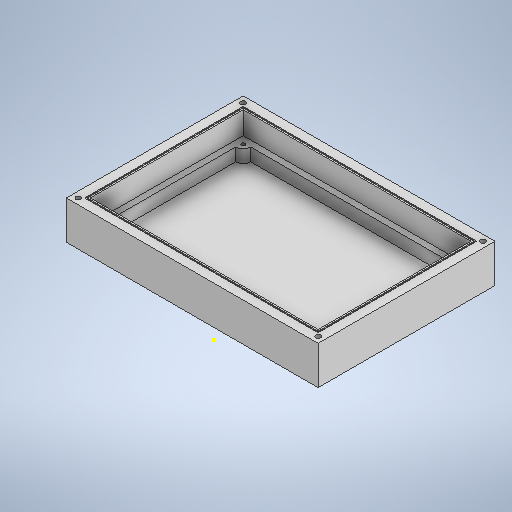
# Autodesk Inventor part: peça pi2
Saved by Autodesk Inventor 2025.1 (Build 291241000, 241)
## iProperties
Created: 2024-10-30
Part Number: peça pi2
Material: Genérico
Document SubType Name: Modeling
Designer: Willi
Density: 1 g/cm^3
Appearance: Padrão
Author: Willi
Autodesk Inventor part; units mm, degrees
ref_plane "YZ Plane" through (0, 0, 0) normal (1, 0, 0) x (0, 1, 0)
ref_plane "XZ Plane" through (0, 0, 0) normal (0, 1, 0) x (-1, 0, 0)
ref_plane "XY Plane" through (0, 0, 0) normal (0, 0, 1) x (1, 0, 0)
sketch "Esboço9" plane through (0, 0, 0) normal (0, 1, 0) x (-1, 0, 0)
  line L0 (123.7607, -142.906) -> (-28.2393, -142.906)
  line L1 (-28.2393, -142.906) -> (-28.2393, -40.906)
  line L2 (-28.2393, -40.906) -> (123.7607, -40.906)
  line L3 (123.7607, -40.906) -> (123.7607, -142.906)
  point P0 (0, 0)
  dimension "d42" = 152
  dimension "d43" = 102
  constraints: 8 end point, 2 parallel, 1 horizontal, 1 perpendicular
  measures "d42" distance of L1.end L2.end
  measures "d43" distance of L0.end L1.end
extrude "Extrusão7" add sketch "Esboço9" along normal blind 10.6
shell "Casca2" thickness 2 removed faces 1 at (-22.4273, 10.6, -74.906)
sketch "Esboço10" plane through (0, 10.6, 0) normal (0, 1, 0) x (1, 0, 0)
  line L0 (-123.7607, 142.906) -> (-123.7607, 40.906) projected
  line L1 (-123.7607, 40.906) -> (28.2393, 40.906) projected
  line L2 (28.2393, 142.906) -> (-123.7607, 142.906) projected
  line L3 (28.2393, 40.906) -> (28.2393, 142.906) projected
  line L4 (-123.7607, 40.906) -> (-131.7607, 40.906)
  line L5 (-131.7607, 40.906) -> (-131.7607, 142.906)
  line L6 (-131.7607, 142.906) -> (-123.7607, 142.906)
  line L7 (-123.7607, 142.906) -> (-123.7607, 40.906)
  line L8 (-131.7607, 142.906) -> (28.2393, 142.906)
  line L9 (28.2393, 142.906) -> (28.2393, 150.906)
  line L10 (28.2393, 150.906) -> (-131.7607, 150.906)
  line L11 (-131.7607, 150.906) -> (-131.7607, 142.906)
  line L12 (28.2393, 40.906) -> (36.2393, 40.906)
  line L13 (36.2393, 40.906) -> (36.2393, 150.906)
  line L14 (36.2393, 150.906) -> (28.2393, 150.906)
  line L15 (28.2393, 150.906) -> (28.2393, 40.906)
  line L16 (-131.7607, 40.906) -> (36.2393, 40.906)
  line L17 (36.2393, 40.906) -> (36.2393, 32.906)
  line L18 (36.2393, 32.906) -> (-131.7607, 32.906)
  line L19 (-131.7607, 32.906) -> (-131.7607, 40.906)
  point P0 (0, 0)
  dimension "d47" = 8
  dimension "d48" = 8
  dimension "d49" = 8
  dimension "d50" = 8
  constraints: 32 end point, 8 parallel, 4 horizontal, 4 perpendicular, 2 point on line
  measures "d47" distance of L5.end L6.end
  measures "d48" distance of L9.end L8.end
  measures "d49" distance of L14.end L13.end
  measures "d50" distance of L16.end L17.end
extrude "Extrusão8" add sketch "Esboço10" along normal blind 15 and the other way blind 10.6 contours L6 L11 L10 L9 L2 | L0 L4 L5 L6 | L1 L12 L17 L18 L19 L4 | L9 L14 L13 L12 L3
sketch "Esboço11" plane through (0, 10.6, 0) normal (0, 1, 0) x (1, 0, 0)
  line L0 (-121.7607, 42.906) -> (-121.7607, 140.906) projected
  line L1 (26.2393, 42.906) -> (-121.7607, 42.906) projected
  line L2 (-121.7607, 140.906) -> (26.2393, 140.906) projected
  line L3 (26.2393, 140.906) -> (26.2393, 42.906) projected
  line L4 (-121.7607, 42.906) -> (-119.7607, 42.906)
  line L5 (-119.7607, 42.906) -> (-119.7607, 140.906)
  line L6 (-119.7607, 140.906) -> (-121.7607, 140.906)
  line L7 (-121.7607, 140.906) -> (-121.7607, 42.906)
  line L8 (26.2393, 140.906) -> (-121.7607, 140.906)
  line L9 (-121.7607, 140.906) -> (-121.7607, 138.906)
  line L10 (-121.7607, 138.906) -> (26.2393, 138.906)
  line L11 (26.2393, 138.906) -> (26.2393, 140.906)
  line L12 (-121.7607, 42.906) -> (26.2393, 42.906)
  line L13 (26.2393, 42.906) -> (26.2393, 44.906)
  line L14 (26.2393, 44.906) -> (-121.7607, 44.906)
  line L15 (-121.7607, 44.906) -> (-121.7607, 42.906)
  line L16 (26.2393, 42.906) -> (24.2393, 42.906)
  line L17 (24.2393, 42.906) -> (24.2393, 140.906)
  line L18 (24.2393, 140.906) -> (26.2393, 140.906)
  line L19 (26.2393, 140.906) -> (26.2393, 42.906)
  point P0 (0, 0)
  point P1 (-119.7607, 138.906)
  point P2 (24.2393, 138.906)
  point P3 (24.2393, 44.906)
  point P4 (-119.7607, 44.906)
  dimension "d55" = 2
  dimension "d56" = 2
  dimension "d57" = 2
  dimension "d58" = 2
  constraints: 32 end point, 8 parallel, 4 horizontal, 4 perpendicular, 4 point on line
  measures "d55" distance of L6.end L5.end
  measures "d56" distance of L9.end L8.end
  measures "d57" distance of L13.end L12.end
  measures "d58" distance of L17.end L18.end
extrude "Extrusão9" add sketch "Esboço11" against normal blind 8.6 contours L0 L14 L5 L1 | L0 L10 L5 L14 | L5 L14 L17 L1 | L0 L2 L5 L10 | L17 L14 L3 L1 | L5 L2 L17 L10 | L17 L10 L3 L14 | L17 L2 L3 L10
sketch "Esboço12" plane through (0, 10.6, 0) normal (0, 1, 0) x (1, 0, 0)
  line L0 (24.2393, 138.906) -> (24.2393, 44.906) projected
  line L1 (24.2393, 44.906) -> (-119.7607, 44.906) projected
  line L2 (-119.7607, 138.906) -> (24.2393, 138.906) projected
  line L3 (-119.7607, 44.906) -> (-119.7607, 138.906) projected
  arc A0 (19.2393, 138.906) -> (24.2393, 133.906) centre (24.2393, 138.906) ccw
  arc A1 (24.2393, 49.906) -> (19.2393, 44.906) centre (24.2393, 44.906) ccw
  arc A2 (-114.7607, 44.906) -> (-119.7607, 49.906) centre (-119.7607, 44.906) ccw
  arc A3 (-119.7607, 133.906) -> (-114.7607, 138.906) centre (-119.7607, 138.906) ccw
  point P0 (0, 0)
  dimension "d61" = 5
  dimension "d62" = 5
  dimension "d63" = 5
  dimension "d64" = 5
  constraints: 8 point on circle, 7 point on line, 4 centre point, 4 coincident
  measures "d61" radius of A0
  measures "d62" radius of A1
  measures "d63" radius of A2
  measures "d64" radius of A3
extrude "Extrusão10" add sketch "Esboço12" against normal blind 8.6 contours L0 A0 L2 | L0 L1 A1 | A3 L3 L2 | L1 L3 A2
sketch "Esboço13" plane through (0, 10.6, 0) normal (0, 1, 0) x (1, 0, 0)
  line L0 (28.2393, 40.906) -> (28.2393, 142.906) projected
  line L1 (-123.7607, 40.906) -> (28.2393, 40.906) projected
  point P0 (0, 0)
  point P1 (23.2393, 45.906)
  dimension "d67" = 5
  dimension "d68" = 5
  measures "d67" distance from line of L0 point (23.239, 45.906)
  measures "d68" distance from line of L1 point (23.239, 45.906)
hole "Furo2" at (23.2393, 10.6, -45.906) direction (0, -1, 0) diameter 2.459 depth 5 tip angle 118 thread size "M3x0.5" class "6H" standard "ISO Metric profile"
sketch "Esboço14" plane through (0, 10.6, 0) normal (0, 1, 0) x (1, 0, 0)
  line L0 (28.2393, 40.906) -> (28.2393, 142.906) projected
  line L1 (28.2393, 142.906) -> (-123.7607, 142.906) projected
  point P0 (0, 0)
  point P1 (23.2393, 137.906)
  dimension "d76" = 5
  dimension "d77" = 5
  measures "d76" distance from line of L0 point (23.239, 137.906)
  measures "d77" distance from line of L1 point (23.239, 137.906)
hole "Furo3" at (23.2393, 10.6, -137.906) direction (0, -1, 0) diameter 2.459 depth 5 tip angle 118 thread size "M3x0.5" class "6H" standard "ISO Metric profile"
sketch "Esboço15" plane through (0, 10.6, 0) normal (0, 1, 0) x (1, 0, 0)
  line L0 (28.2393, 142.906) -> (-123.7607, 142.906) projected
  line L1 (-123.7607, 142.906) -> (-123.7607, 40.906) projected
  point P0 (0, 0)
  point P1 (-118.7607, 137.906)
  dimension "d85" = 5
  dimension "d86" = 5
  measures "d85" distance from line of L0 point (-118.761, 137.906)
  measures "d86" distance from line of L1 point (-118.761, 137.906)
hole "Furo4" at (-118.7607, 10.6, -137.906) direction (0, -1, 0) diameter 2.459 depth 5 tip angle 118 thread size "M3x0.5" class "6H" standard "ISO Metric profile"
sketch "Esboço16" plane through (0, 10.6, 0) normal (0, 1, 0) x (1, 0, 0)
  line L0 (-123.7607, 142.906) -> (-123.7607, 40.906) projected
  line L1 (-123.7607, 40.906) -> (28.2393, 40.906) projected
  point P0 (0, 0)
  point P1 (-118.7607, 45.906)
  dimension "d94" = 5
  dimension "d95" = 5
  measures "d94" distance from line of L0 point (-118.761, 45.906)
  measures "d95" distance from line of L1 point (-118.761, 45.906)
hole "Furo5" at (-118.7607, 10.6, -45.906) direction (0, -1, 0) diameter 2.459 depth 5 tip angle 118 thread size "M3x0.5" class "6H" standard "ISO Metric profile"
sketch "Esboço18" plane through (0, 25.6, 0) normal (0, 1, 0) x (1, 0, 0)
  point P0 (0, 0)
sketch "Esboço19" plane through (0, 25.6, 0) normal (0, 1, 0) x (1, 0, 0)
  point P0 (0, 0)
sketch "Esboço20" plane through (0, 25.6, 0) normal (0, 1, 0) x (1, 0, 0)
  line L0 (-131.7607, 32.906) -> (36.2393, 32.906) projected
  line L1 (-131.7607, 150.906) -> (-131.7607, 32.906) projected
  point P0 (0, 0)
  point P1 (-127.7607, 36.906)
  dimension "d104" = 4
  dimension "d105" = 4
  measures "d104" distance from line of L0 point (-127.761, 36.906)
  measures "d105" distance from line of L1 point (-127.761, 36.906)
hole "Furo6" at (-127.7607, 25.6, -36.906) direction (0, -1, 0) diameter 3.242 depth 15 tip angle 118 thread size "M4x0.7" class "6H" standard "ISO Metric profile"
sketch "Esboço21" plane through (0, 25.6, 0) normal (0, 1, 0) x (1, 0, 0)
  line L0 (28.2393, 142.906) -> (28.2393, 40.906) projected
  line L1 (-124.3607, 143.906) -> (28.8393, 143.906)
  line L2 (29.2393, 143.506) -> (29.2393, 40.306)
  line L3 (28.8393, 39.906) -> (-124.3607, 39.906)
  line L4 (-124.7607, 40.306) -> (-124.7607, 143.506)
  line L5 (-125.2607, 39.006) -> (29.7393, 39.006)
  line L6 (30.1393, 39.406) -> (30.1393, 144.406)
  line L7 (29.7393, 144.806) -> (-125.2607, 144.806)
  line L8 (-125.6607, 144.406) -> (-125.6607, 39.406)
  arc A0 (-125.6607, 39.406) -> (-125.2607, 39.006) centre (-125.2607, 39.406) ccw
  arc A1 (-124.7607, 40.306) -> (-124.3607, 39.906) centre (-124.3607, 40.306) ccw
  arc A2 (-124.3607, 143.906) -> (-124.7607, 143.506) centre (-124.3607, 143.506) ccw
  arc A3 (-125.2607, 144.806) -> (-125.6607, 144.406) centre (-125.2607, 144.406) ccw
  arc A4 (28.8393, 39.906) -> (29.2393, 40.306) centre (28.8393, 40.306) ccw
  arc A5 (29.7393, 39.006) -> (30.1393, 39.406) centre (29.7393, 39.406) ccw
  arc A6 (29.2393, 143.506) -> (28.8393, 143.906) centre (28.8393, 143.506) ccw
  arc A7 (30.1393, 144.406) -> (29.7393, 144.806) centre (29.7393, 144.406) ccw
  point P0 (0, 0)
  point P1 (-123.7607, 40.906)
  dimension "d117" = 0.9
  dimension "d118" = 0.4
  constraints: 16 end point, 16 point on circle, 16 tangent, 8 centre point, 7 equal radius, 4 parallel, 2 perpendicular, 3 other
  measures "d117" distance between parallel lines of L3 L5
  measures "d118" radius of A0
extrude "Extrusão11" cut sketch "Esboço21" against normal blind 0.6
sketch "Esboço22" plane through (0, 25.6, 0) normal (0, 1, 0) x (1, 0, 0)
  line L0 (-131.7607, 150.906) -> (-131.7607, 32.906) projected
  line L1 (36.2393, 150.906) -> (-131.7607, 150.906) projected
  line L2 (36.2393, 32.906) -> (36.2393, 150.906) projected
  line L3 (-131.7607, 32.906) -> (36.2393, 32.906) projected
  point P0 (0, 0)
  point P1 (-127.7607, 146.906)
  point P2 (32.2393, 146.906)
  point P3 (32.2393, 36.906)
  dimension "d121" = 4
  dimension "d122" = 4
  dimension "d123" = 4
  dimension "d124" = 4
  dimension "d125" = 4
  dimension "d126" = 4
  measures "d121" distance from line of L0 point (-127.761, 146.906)
  measures "d122" distance from line of L1 point (-127.761, 146.906)
  measures "d123" distance from line of L2 point (32.239, 146.906)
  measures "d124" distance from line of L1 point (32.239, 146.906)
  measures "d125" distance from line of L2 point (32.239, 36.906)
  measures "d126" distance from line of L3 point (32.239, 36.906)
hole "Furo7" at (-127.7607, 25.6, -146.906) at (32.2393, 25.6, -146.906) at (32.2393, 25.6, -36.906) direction (0, -1, 0) diameter 3.242 depth 15 tip angle 118 thread size "M4x0.7" class "6H" standard "ISO Metric profile"
